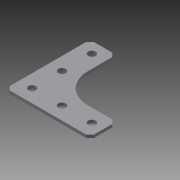
# Autodesk Inventor part: 3x3 Gusset
Saved by Autodesk Inventor 2014 (Build 180170000, 170)
## iProperties
Created: 2015-01-29
Part Number: 3x3 Gusset
Material: Generic
Document SubType Name: Sheet Metal
Designer: chappelled
Density: 1 g/cm^3
Appearance: Default
Sheet Metal Rule: Default
Author: chappelled
Autodesk Inventor part; units mm, degrees
ref_plane "YZ Plane" through (0, 0, 0) normal (1, 0, 0) x (0, 1, 0)
ref_plane "XZ Plane" through (0, 0, 0) normal (0, 1, 0) x (-1, 0, 0)
ref_plane "XY Plane" through (0, 0, 0) normal (0, 0, 1) x (1, 0, 0)
sketch "Sketch1" plane through (0, 0, 0) normal (0, 1, 0) x (-1, 0, 0)
  line L0 (-3.175, 0) -> (-19.05, 0)
  line L1 (-71.4375, 52.3875) -> (-71.4375, 68.2625)
  line L2 (-68.2625, 71.4375) -> (-3.175, 71.4375)
  line L3 (0, 68.2625) -> (0, 3.175)
  line L4 (-3.175, 0) -> (0, 3.175)
  line L5 (0, 68.2625) -> (-3.175, 71.4375)
  line L6 (-68.2625, 71.4375) -> (-71.4375, 68.2625)
  line L7 (-22.225, 3.175) -> (-22.225, 23.8125)
  line L8 (-47.625, 49.2125) -> (-68.2625, 49.2125)
  arc A0 (-22.225, 23.8125) -> (-47.625, 49.2125) centre (-47.625, 23.8125) ccw
  line L9 (-22.225, 3.175) -> (-19.05, 0)
  line L10 (-71.4375, 52.3875) -> (-68.2625, 49.2125)
  point P0 (0, 0)
  point P1 (-71.4375, 71.4375)
  point P2 (0, 71.4375)
  point P3 (-22.225, 49.2125)
  point P4 (-22.225, 0)
  point P5 (-71.4375, 49.2125)
  dimension "d0" = 71.4375
  dimension "d2" = 3.175
  dimension "d3" = 3.175
  dimension "d4" = 3.175
  dimension "d5" = 3.175
  dimension "d6" = 3.175
  dimension "d7" = 3.175
  dimension "d11" = 3.175
  dimension "d12" = 3.175
  dimension "d13" = 3.175
  dimension "d14" = 3.175
  dimension "d32" = 15.875
  dimension "d35" = 15.875
  dimension "d37" = 71.4375
  dimension "d38" = 25.4
  dimension "d39" = 47.625
  dimension "d40" = 47.625
  constraints: 22 end point, 12 point on line, 2 parallel, 2 point on circle, 2 tangent, 1 centre point, 1 horizontal, 1 perpendicular
  measures "d0" distance of point (-71.438, 71.437) point (0, 71.438)
  measures "d2" distance of L0.start point (0, 0)
  measures "d3" distance of L3.end point (0, 0)
  measures "d4" distance of L3.start point (0, 71.438)
  measures "d5" distance of L2.end point (0, 71.438)
  measures "d6" distance of L2.start point (-71.438, 71.437)
  measures "d7" distance of L1.end point (-71.438, 71.437)
  measures "d11" distance of L7.start point (-22.225, 0)
  measures "d12" distance of L0.end point (-22.225, 0)
  measures "d13" distance of L1.start point (-71.438, 49.212)
  measures "d14" distance of L8.end point (-71.438, 49.212)
  measures "d32" distance of L1.start L1.end
  measures "d35" distance of L0.start L0.end
  measures "d37" distance between parallel lines of L0 L2
  measures "d38" radius of A0
  measures "d39" distance from line of L3 A0.centre
  measures "d40" distance from line of L2 A0.centre
extrude "Extrusion1" add sketch "Sketch1" along normal blind 2.54
hole "Hole1" at (11.1125, 2.54, 60.325) direction (0, -1, 0) diameter 6.35 end through all
pattern_linear "Rectangular Pattern1" count 3 spacing 25.4 along (0, 0, -1) of "Hole1"
pattern_linear "Rectangular Pattern2" count 3 spacing 25.4 along (1, 0, 0) of "Hole1"
equation "\"d3\" = d2"
equation "\"d4\" = d2"
equation "\"d5\" = d4"
equation "\"d6\" = d2"
equation "\"d7\" = d6"
equation "\"d12\" = d11"
equation "\"d13\" = d11"
equation "\"d14\" = d13"
equation "\"d35\" = d32"
equation "\"d37\" = d0"
equation "\"d40\" = d39"
equation "\"BendRadius\" = Thickness"
equation "\"BendReliefWidth\" = Thickness"
equation "\"BendReliefDepth\" = 0.5 * Thickness"
equation "\"CornerReliefSize\" = 4 * Thickness"
equation "\"MinimumRemnant\" = 2 * Thickness"
equation "\"TransitionRadius\" = BendRadius"
equation "\"JacobiRadiusSize\" = Thickness"
equation "\"GapSize\" = Thickness"
equation "\"Thickness\" = 3.048"
body "Solid1"
